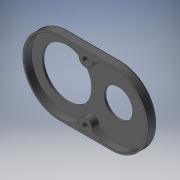
# Autodesk Inventor part: AA041
Saved by Autodesk Inventor 2017 SP1 (Build 210196100, 196)
## iProperties
Created: 2018-01-23
Part Number: AA041
Material: ABS Plastic
Document SubType Name: Modeling
Designer: Zach
Density: 1.06 g/cm^3
Appearance: CR White
Author: Zach
Autodesk Inventor part; units mm, degrees
ref_plane "YZ Plane" through (0, 0, 0) normal (1, 0, 0) x (0, 1, 0)
ref_plane "XZ Plane" through (0, 0, 0) normal (0, 1, 0) x (-1, 0, 0)
ref_plane "XY Plane" through (0, 0, 0) normal (0, 0, 1) x (1, 0, 0)
sketch "Sketch1" plane through (0, 0, 0) normal (0, 0, 1) x (1, 0, 0)
  circle A0 centre (0, 0) radius 20 construction
  circle A1 centre (27, 0) radius 20 construction
  line L0 (0, 20) -> (27, 20)
  line L1 (0, -20) -> (27, -20)
  arc A2 (27, -20) -> (27, 20) centre (27, 0) ccw
  arc A3 (0, 20) -> (0, -20) centre (0, 0) ccw
  circle A4 centre (13.5, 15) radius 1.5
  circle A5 centre (13.5, -15) radius 1.5
  point P0 (13.5, 20)
  point P1 (13.5, -20)
  dimension "d0" = 40
  dimension "d1" = 40
  dimension "d2" = 27
  dimension "d5" = 3
  dimension "d6" = 3
  dimension "d7" = 5
  dimension "d8" = 5
  constraints: 8 point on circle, 6 centre point, 6 tangent, 4 end point, 2 midpoint, 2 vertical alignment, 1 coincident, 1 concentric, 1 horizontal alignment
  measures "d0" diameter of A0
  measures "d1" diameter of A1
  measures "d2" distance of A1.centre point (0, 0)
  measures "d5" diameter of A4
  measures "d6" diameter of A5
  measures "d7" distance from line of L0 A4.centre
  measures "d8" distance from line of A5.centre L1
extrude "Extrusion1" add sketch "Sketch1" along normal blind 1
sketch "Sketch2" plane through (0, 0, 1) normal (0, 0, 1) x (1, 0, 0)
  arc A0 (0, 20) -> (0, -20) centre (0, 0) ccw projected
  arc A1 (27, -20) -> (27, 20) centre (27, 0) ccw projected
  circle A2 centre (0, 0) radius 18.5 construction
  circle A3 centre (27, 0) radius 18.5 construction
  line L0 (27, 20) -> (0, 20) projected
  arc A4 (13.5, 12.6491) -> (0, 18.5) centre (0, 0) ccw
  arc A5 (27, 18.5) -> (13.5, 12.6491) centre (27, 0) ccw
  arc A6 (0, -18.5) -> (13.5, -12.6491) centre (0, 0) ccw
  arc A7 (13.5, -12.6491) -> (27, -18.5) centre (27, 0) ccw
  line L1 (0, -20) -> (27, -20) projected
  circle A8 centre (13.5, -15) radius 1.5 projected
  circle A9 centre (13.5, 15) radius 1.5 projected
  arc A10 (0, 18.5) -> (0, -18.5) centre (0, 0) ccw
  arc A11 (27, -18.5) -> (27, 18.5) centre (27, 0) ccw
  circle A12 centre (13.5, -15) radius 3.5
  circle A13 centre (13.5, 15) radius 3.5
  point P0 (0, 0)
  dimension "d9" = 37
  dimension "d10" = 37
  dimension "d26" = 7
  dimension "d27" = 7
  constraints: 20 point on circle, 10 centre point, 9 concentric, 4 coincident, 2 vertical alignment
  measures "d9" diameter of A2
  measures "d10" diameter of A3
  measures "d26" diameter of A12
  measures "d27" diameter of A13
extrude "Extrusion2" add sketch "Sketch2" along normal blind 3.8 contours L0 A1 L1 A0 | A5 A13 A4 | A4 A13 A5 | A12 A7 A6 | A6 A7 A12
sketch "Sketch3" plane through (0, 0, 0) normal (0, 0, -1) x (-1, 0, 0)
  circle A0 centre (0, 0) radius 13
  arc A1 (-27, 20) -> (-27, -20) centre (-27, 0) ccw projected
  circle A2 centre (-27, 0) radius 7.5
  dimension "d13" = 26
  dimension "d28" = 15
  constraints: 2 centre point, 2 coincident
  measures "d13" diameter of A0
  measures "d28" diameter of A2
extrude "Extrusion3" cut sketch "Sketch3" against normal through all
sketch "Sketch4" plane through (0, 0, 0) normal (0, 0, -1) x (-1, 0, 0)
  circle A0 centre (0, 0) radius 13 construction
  circle A1 centre (-13.5, -15) radius 1.5 construction
  circle A2 centre (-13.5, 15) radius 1.5 construction
  line L0 (0, 20) -> (-27, 20) projected
  arc A3 (-27, 20) -> (-27, -20) centre (-27, 0) ccw projected
  line L1 (-27, -20) -> (0, -20) projected
  arc A4 (0, -20) -> (0, 20) centre (0, 0) ccw projected
  line L2 (0, -19.4) -> (-27, -19.4)
  arc A5 (-27, 19.4) -> (-27, -19.4) centre (-27, 0) ccw
  line L3 (-27, 19.4) -> (0, 19.4)
  arc A6 (0, -19.4) -> (0, 19.4) centre (0, 0) ccw
  dimension "d16" = 0.6
  constraints: 4 end point, 4 point on circle, 2 centre point, 3 other
  measures "d16" distance between parallel lines of L1 L2
extrude "Extrusion4" cut sketch "Sketch4" against normal through all
sketch "Sketch7" plane through (0, 0, 0) normal (0, 0, -1) x (-1, 0, 0)
  circle A0 centre (-13.5, -15) radius 1.5 projected
  circle A1 centre (-13.5, 15) radius 1.5 projected
  circle A2 centre (-13.5, -15) radius 3
  circle A3 centre (-13.5, 15) radius 3
  point P0 (0, 0)
  dimension "d22" = 6
  dimension "d23" = 6
  constraints: 2 centre point, 2 coincident
  measures "d22" diameter of A2
  measures "d23" diameter of A3
extrude "Extrusion5" cut sketch "Sketch7" against normal blind 3 contours A0 | A1 | A2 | A3
fillet "Fillet1" radius 1 4 edges at (13.5, 19.4, 0) (46.4, 0, 0) (13.5, -19.4, 0) (-19.4, 0, 0)
body "Solid1"
